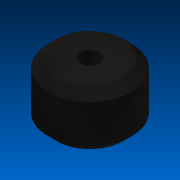
# Autodesk Inventor part: Omron SS-01GL2-E Microswitch Roller
Saved by Autodesk Inventor 2013 (Build 170138000, 138)
## iProperties
Created: 2012-05-23
Material: Acetal Resin, Black
Document SubType Name: Modeling
Designer: sdarley
Density: 1 g/cm^3
Project: Microswitch - Omron SS-01GL2-E
Description: Omron SS-01GL2-E Microswitch Roller
Author: sdarley
Title: Omron SS-01GL2-E Microswitch Roller
Revision Number: 1
Autodesk Inventor part; units mm, degrees
ref_plane "YZ Plane" through (0, 0, 0) normal (1, 0, 0) x (0, 1, 0)
ref_plane "XZ Plane" through (0, 0, 0) normal (0, 1, 0) x (-1, 0, 0)
ref_plane "XY Plane" through (0, 0, 0) normal (0, 0, 1) x (1, 0, 0)
sketch "Sketch1" plane through (0, 0, 0) normal (0, 0, 1) x (1, 0, 0)
  circle A0 centre (0, 0) radius 2.4
  circle A1 centre (0, 0) radius 0.55
  dimension "d0" = 4.8
  dimension "d1" = 1.1
  constraints: 2 centre point, 2 coincident
  measures "d0" diameter of A0
  measures "d1" diameter of A1
extrude "Extrusion1" add sketch "Sketch1" along normal mid plane 3.2
chamfer "Chamfer1" distance 0.5 angle 45 2 edges at (-2.4, 0, -1.6) (-2.4, 0, 1.6)
body "Solid1"
